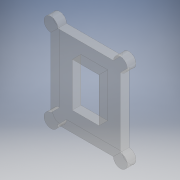
# Autodesk Inventor part: cubierta2
Saved by Autodesk Inventor 2016 (Build 200138000, 138)
## iProperties
Created: 2017-05-08
Part Number: cubierta2
Material: Generic
Document SubType Name: Modeling
Designer: rdiaz
Density: 1 g/cm^3
Appearance: Polycarbonate - Clear
Author: rdiaz
Autodesk Inventor part; units mm, degrees
ref_plane "YZ Plane" through (0, 0, 0) normal (1, 0, 0) x (0, 1, 0)
ref_plane "XZ Plane" through (0, 0, 0) normal (0, 1, 0) x (-1, 0, 0)
ref_plane "XY Plane" through (0, 0, 0) normal (0, 0, 1) x (1, 0, 0)
sketch "Sketch1" plane through (0, 0, 0) normal (0, 1, 0) x (-1, 0, 0)
  line L0 (12.7, 7.7) -> (-12.7, 7.7)
  line L1 (-12.7, 7.7) -> (-12.7, -7.7)
  line L2 (-12.7, -7.7) -> (12.7, -7.7)
  line L3 (12.7, -7.7) -> (12.7, 7.7)
  line L4 (24, -20) -> (-24, -20)
  line L5 (-24, -20) -> (-24, 20)
  line L6 (-24, 20) -> (24, 20)
  line L7 (24, 20) -> (24, -20)
  circle A0 centre (24, -20) radius 4
  circle A1 centre (-24, -20) radius 4
  circle A2 centre (24, 20) radius 4
  circle A3 centre (-24, 20) radius 4
  point P0 (0, 0)
  point P1 (0, -7.7)
  point P2 (12.7, 0)
  point P3 (0, 20)
  point P4 (24, 0)
  dimension "d0" = 25.4
  dimension "d1" = 15.4
  dimension "d11" = 8
  dimension "d12" = 8
  dimension "d13" = 8
  dimension "d14" = 8
  dimension "d15" = 40
  dimension "d16" = 48
  constraints: 16 end point, 4 centre point, 4 coincident, 4 midpoint, 4 parallel, 2 horizontal, 2 horizontal alignment, 2 perpendicular, 2 vertical alignment
  measures "d0" distance of L1.end L2.end
  measures "d1" distance of L2.end L0.start
  measures "d11" diameter of A0
  measures "d12" diameter of A1
  measures "d13" diameter of A2
  measures "d14" diameter of A3
  measures "d15" distance between parallel lines of L6 L4
  measures "d16" distance between parallel lines of L5 L7
extrude "Extrusion1" add sketch "Sketch1" along normal blind 5
fillet "Fillet1" [suppressed]
body "Solid1"
